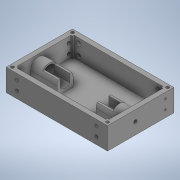
# Autodesk Inventor part: BodyWedgeBaseV3.1
Saved by Autodesk Inventor 2020 (Build 240168000, 168)
## iProperties
Created: 2023-11-26
Part Number: BodyWedgeBaseV3.1
Material: H TPU
Document SubType Name: Modeling
Designer: smz3rm
Density: 0.941117 g/cm^3
Appearance: Generic
Mass: 101.073 g
Surface Area: 496.603 cm^2
Volume: 107.397 cm^3
SideThickness: 6.000 mm
BaseThickness: 3.000 mm
TopThickness: 1.778 mm
BoxWidth: 130.000 mm
BoxLength: 85.000 mm
Height: 30.000 mm
DriveMotorHeight: 15.000 mm
DriveMotorMountThickness: 2.000 mm
DriveMotorOffset: 49.500 mm
DriveMotorDia: 16.500 mm
SideArmorWidth: 15.000 mm
ForkLength: 80.000 mm
WheelWidth: 16.510 mm
DriveMotorHoleDia: 4.200 mm
ForkPlugDia: 4.000 mm
ForkPlugTolerance: 0.750 mm
ForkPlugLength: 8.000 mm
M2ScrewInsertDia: 2.900 mm
M2ScrewInsertDepth: 7.000 mm
M3ScrewHeadDia: 6.100 mm
M3ScrewDia: 3.100 mm
M3ScrewHeadDepth: 2.300 mm
M3ScrewInsertDia: 4.000 mm
M3ScrewInsertDepth: 7.000 mm
M2ScrewHeadDia: 4.000 mm
M2ScrewHeadDepth: 2.200 mm
M2ScrewDia: 2.200 mm
M3ScrewInsertBrim: 8.000 mm
ForkScrewOffset: 8.000 mm
SideScrewVerticalOffset: 6.000 mm
RearScrewHorizontalOffset: 14.000 mm
SideScrewHorizontalOffset: 11.000 mm
M3ScrewHeadTaper: -32.50 deg
Author: smz3rm
Autodesk Inventor part; units mm, degrees
ref_plane "YZ Plane" through (0, 0, 0) normal (1, 0, 0) x (0, 1, 0)
ref_plane "XZ Plane" through (0, 0, 0) normal (0, 1, 0) x (-1, 0, 0)
ref_plane "XY Plane" through (0, 0, 0) normal (0, 0, 1) x (1, 0, 0)
sketch "Sketch1" plane through (0, 0, 0) normal (0, 1, 0) x (-1, 0, 0)
  line L0 (65, 42.5) -> (-65, 42.5)
  line L1 (-65, 42.5) -> (-65, -42.5)
  line L2 (-65, -42.5) -> (65, -42.5)
  line L3 (65, -42.5) -> (65, 42.5)
  line L4 (65, 42.5) -> (-65, -42.5) construction
  line L5 (-65, 42.5) -> (65, -42.5) construction
  line L6 (0, -56) -> (0, 56) projected
  point P0 (0, 0)
  dimension "d0" = 130
  dimension "d1" = 85
  constraints: 12 end point, 2 midpoint, 2 parallel, 1 horizontal, 1 perpendicular
  measures "d0" distance of L2.end L1.end
  measures "d1" distance of L1.end L0.end
sketch "Sketch1 outline for Extrusion1" plane through (0, 0, 0) normal (0, 1, 0) x (-1, 0, 0)
  line L0 (65, -42.5) -> (65, 42.5)
  line L1 (-65, -42.5) -> (65, -42.5)
  line L2 (-65, 42.5) -> (-65, -42.5)
  line L3 (65, 42.5) -> (-65, 42.5)
extrude "Extrusion1" add sketch "Sketch1 outline for Extrusion1" along normal blind 3
sketch "Sketch2" plane through (0, 3, 0) normal (0, 1, 0) x (1, 0, 0)
  line L0 (-65, 42.5) -> (-65, -42.5) projected
  line L1 (-65, -42.5) -> (65, -42.5) projected
  line L2 (65, -42.5) -> (65, 42.5) projected
  line L3 (59, -36.5) -> (-59, -36.5)
  line L4 (-59, -36.5) -> (-59, 36.5)
  line L5 (-59, 36.5) -> (59, 36.5)
  line L6 (59, 36.5) -> (59, -36.5)
  line L7 (59, -36.5) -> (-59, 36.5) construction
  line L8 (-59, -36.5) -> (59, 36.5) construction
  line L9 (65, 42.5) -> (-65, 42.5) projected
  line L10 (-65, -42.5) -> (65, -42.5) projected
  line L11 (65, -42.5) -> (57, -42.5)
  line L12 (57, -42.5) -> (57, -34.5)
  line L13 (57, -34.5) -> (65, -34.5)
  line L14 (65, -34.5) -> (65, -42.5)
  line L15 (-65, -42.5) -> (-57, -42.5)
  line L16 (-57, -42.5) -> (-57, -34.5)
  line L17 (-57, -34.5) -> (-65, -34.5)
  line L18 (-65, -34.5) -> (-65, -42.5)
  line L19 (65, 42.5) -> (-65, 42.5) projected
  line L20 (-65, 42.5) -> (-57, 42.5)
  line L21 (-57, 42.5) -> (-57, 34.5)
  line L22 (-57, 34.5) -> (-65, 34.5)
  line L23 (-65, 34.5) -> (-65, 42.5)
  line L24 (65, 42.5) -> (57, 42.5)
  line L25 (57, 42.5) -> (57, 34.5)
  line L26 (57, 34.5) -> (65, 34.5)
  line L27 (65, 34.5) -> (65, 42.5)
  point P0 (0, 0)
  point P1 (59, 34.5)
  point P2 (57, 36.5)
  point P3 (-59, 34.5)
  point P4 (-57, 36.5)
  point P5 (-59, -34.5)
  point P6 (-57, -36.5)
  point P7 (59, -34.5)
  point P8 (57, -36.5)
  dimension "d36" = 118
  dimension "d37" = 73
  dimension "d173" = 8
  dimension "d176" = 8
  dimension "d177" = 8
  dimension "d178" = 8
  constraints: 44 end point, 10 parallel, 9 perpendicular, 5 horizontal, 2 midpoint
  measures "d36" distance of L4.end L5.end
  measures "d37" distance between parallel lines of L5 L3
  measures "d173" distance of L12.end L13.end
  measures "d176" distance of L15.end L16.end
  measures "d177" distance of L21.end L22.end
  measures "d178" distance of L25.end L26.end
sketch "Sketch2 outline for Extrusion2" plane through (0, 3, 0) normal (0, 1, 0) x (1, 0, 0)
  line L0 (65, 42.5) -> (-65, 42.5)
  line L1 (-65, 42.5) -> (-65, -42.5)
  line L2 (-65, -42.5) -> (65, -42.5)
  line L3 (65, -42.5) -> (65, 42.5)
  line L4 (59, 34.5) -> (59, -34.5)
  line L5 (59, -34.5) -> (57, -34.5)
  line L6 (57, -34.5) -> (57, -36.5)
  line L7 (57, -36.5) -> (-57, -36.5)
  line L8 (-57, -36.5) -> (-57, -34.5)
  line L9 (-57, -34.5) -> (-59, -34.5)
  line L10 (-59, -34.5) -> (-59, 34.5)
  line L11 (-59, 34.5) -> (-57, 34.5)
  line L12 (-57, 34.5) -> (-57, 36.5)
  line L13 (-57, 36.5) -> (57, 36.5)
  line L14 (57, 36.5) -> (57, 34.5)
  line L15 (57, 34.5) -> (59, 34.5)
extrude "Extrusion2" add sketch "Sketch2 outline for Extrusion2" along normal blind 25.222
sketch "Sketch7" plane through (-59, 3, 36.5) normal (1, 0, 0) x (0, 0, -1)
  circle A0 centre (29.5, 12) radius 8.25
  line L0 (79, -3) -> (-6, -3) projected
  circle A1 centre (29.5, 12) radius 10.25
  line L1 (19.25, 12) -> (39.75, 12)
  line L2 (39.75, 12) -> (39.75, 0)
  line L3 (-6, -3) -> (-6, 25.222) projected
  line L4 (19.25, 12) -> (19.25, 0)
  line L5 (71, 0) -> (2, 0) projected
  line L6 (79, -3) -> (-6, -3) projected
  line L7 (-6, -3) -> (-6, 25.222) projected
  line L8 (79, 25.222) -> (-6, 25.222) projected
  line L9 (79, -3) -> (79, 25.222) projected
  line L10 (79, -3) -> (79, 25.222) projected
  point P0 (36.5, -3)
  point P1 (0, 0)
  point P2 (54, -3)
  point P3 (68, 0)
  point P4 (21.25, 12)
  point P5 (37.75, 12)
  dimension "MotorDiameter" = 16.5
  dimension "d18" = 15
  dimension "d20" = 2
  dimension "d183" = 49.5
  constraints: 6 end point, 2 centre point, 2 point on circle, 2 vertical, 1 horizontal, 1 point on line, 1 tangent
  measures "MotorDiameter" diameter of A0
  measures "d18" distance from line of L0 A0.centre
  measures "d20" radial gap between concentric circles of A0 A1
  measures "d183" distance from line of L10 A0.centre
sketch "Sketch7 outline for Extrusion5" plane through (-59, 3, 36.5) normal (1, 0, 0) x (0, 0, -1)
  circle A0 centre (29.5, 12) radius 8.25
  arc A1 (39.75, 12) -> (19.25, 12) centre (29.5, 12) ccw
  line L0 (19.25, 12) -> (19.25, 0)
  line L1 (19.25, 0) -> (39.75, 0)
  line L2 (39.75, 0) -> (39.75, 12)
extrude "Extrusion5" add sketch "Sketch7 outline for Extrusion5" along normal blind 14
sketch "Sketch8" plane through (-45, 3, 36.5) normal (1, 0, 0) x (0, 0, -1)
  arc A0 (39.75, 12) -> (19.25, 12) centre (29.5, 12) ccw
  arc A1 (39.75, 12) -> (19.25, 12) centre (29.5, 12) ccw
  arc A2 (21.25, 12) -> (21.25, 12) centre (29.5, 12) ccw
  line L0 (39.75, 0) -> (19.25, 0)
  circle A3 centre (29.5, 12) radius 7.75
  line L1 (23.4, 17.554503) -> (23.4, 0)
  line L2 (29.5, 19.75) -> (29.5, 4.25)
  line L3 (35.6, 17.554503) -> (35.6, 0)
  circle A4 centre (29.5, 12) radius 8.25
  arc A5 (39.75, 12) -> (19.25, 12) centre (29.5, 12) ccw
  line L4 (35.6, 17.554503) -> (38.114523, 17.554503)
  line L5 (23.4, 17.554503) -> (20.885477, 17.554503)
  line L6 (19.25, 12) -> (19.25, 0)
  line L7 (39.75, 0) -> (19.25, 0)
  line L8 (39.75, 0) -> (39.75, 12)
  line L9 (19.25, 12) -> (19.25, 0)
  line L10 (39.75, 0) -> (19.25, 0)
  line L11 (39.75, 0) -> (39.75, 12)
  point P0 (36.5, -3)
  point P1 (19.25, 12)
  point P2 (44.75, 12)
  point P3 (35.6, 7.219571)
  point P4 (23.4, 7.219571)
  point P5 (20.885477, 17.554503)
  point P6 (39.75, 12)
  point P7 (35.6, 16.780429)
  point P8 (23.4, 16.780429)
  point P9 (19.25, 12)
  point P10 (19.25, 0)
  dimension "d145" = 15.5
  dimension "d146" = 15.5
  dimension "d147" = 12.2
  constraints: 10 end point, 4 point on circle, 2 horizontal, 2 symmetric about line, 1 centre point, 1 coincident, 1 perpendicular, 1 vertical, 2 other
  measures "d145" diameter of A3
  measures "d146" distance of L2.start L2.end
  measures "d147" distance between parallel lines of L1 L3
sketch "Sketch8 outline for Extrusion6" plane through (-45, 3, 36.5) normal (1, 0, 0) x (0, 0, -1)
  line L0 (39.75, 0) -> (39.75, 12)
  arc A0 (39.75, 12) -> (38.114523, 17.554503) centre (29.5, 12) ccw
  line L1 (38.114523, 17.554503) -> (35.6, 17.554503)
  line L2 (35.6, 17.554503) -> (35.6, 7.219571)
  arc A1 (35.6, 7.219571) -> (23.4, 7.219571) centre (29.5, 12) cw
  line L3 (23.4, 7.219571) -> (23.4, 17.554503)
  line L4 (23.4, 17.554503) -> (20.885477, 17.554503)
  arc A2 (20.885477, 17.554503) -> (19.25, 12) centre (29.5, 12) ccw
  line L5 (19.25, 12) -> (19.25, 0)
  line L6 (19.25, 0) -> (39.75, 0)
extrude "Extrusion6" add sketch "Sketch8 outline for Extrusion6" along normal blind 20
sketch "Sketch9" plane through (-59, 17, 13) normal (1, 0, 0) x (0, 0, -1)
  line L0 (55.5, -17) -> (-29.5, -17)
  line L1 (-29.5, -17) -> (-29.5, 11.222)
  arc A0 (-0.1, 3.554503) -> (12.1, 3.554503) centre (6, -2) ccw
  circle A1 centre (6, -2) radius 8.25
  circle A2 centre (6, -2) radius 2.1
  arc A3 (12.1, 3.554503) -> (-0.1, 3.554503) centre (6, -2) ccw
  point P0 (13, -17)
  point P1 (44, -20)
  dimension "d148" = 4.2
  constraints: 1 centre point, 1 coincident, 1 other
  measures "d148" diameter of A2
sketch "Sketch9 outline for Extrusion7" plane through (-59, 17, 13) normal (1, 0, 0) x (0, 0, -1)
  circle A0 centre (6, -2) radius 2.1
extrude "Extrusion7" cut sketch "Sketch9 outline for Extrusion7" against normal up to surface (6 mm away)
mirror "Mirror2" about plane through (0, 0, 0) normal (1, 0, 0) of "Extrusion7", "Extrusion6", "Extrusion5"
sketch "Sketch28" plane through (-59, 3, -36.5) normal (0, 0, 1) x (1, 0, 0)
  line L0 (116, 0) -> (2, 0) projected
  line L1 (110, 19) -> (110, 5)
  line L2 (110, 5) -> (8, 5)
  line L3 (8, 5) -> (8, 19)
  line L4 (8, 19) -> (110, 19)
  circle A0 centre (8, 19) radius 3.05
  circle A1 centre (8, 5) radius 3.05
  circle A2 centre (110, 19) radius 3.05
  circle A3 centre (110, 5) radius 3.05
  line L5 (2, 25.222) -> (116, 25.222) projected
  line L6 (116, 0) -> (116, 25.222) projected
  line L7 (2, 0) -> (2, 25.222) projected
  line L8 (0, 0) -> (0, 25.222) projected
  line L9 (0, 0) -> (0, 25.222) projected
  line L10 (118, 0) -> (118, 25.222) projected
  line L11 (118, 0) -> (118, 25.222) projected
  line L12 (0, 14.1) -> (0, 9.9) projected
  line L13 (118, 9.9) -> (118, 14.1) projected
  line L14 (0, 12) -> (0, 12) projected
  line L15 (118, 12) -> (118, 12) projected
  line L16 (0, 0) -> (0, 12) projected
  line L17 (0, 12) -> (0, 0) projected
  line L18 (118, 12) -> (118, 0) projected
  line L19 (118, 0) -> (118, 12) projected
  point P0 (59, -3)
  point P1 (0, 22.25)
  point P2 (0, 1.75)
  point P3 (118, 22.25)
  point P4 (118, 1.75)
  dimension "d120" = 6.1
  dimension "d121" = 6.1
  dimension "d122" = 6.1
  dimension "d123" = 6.1
  dimension "d132" = 6.222
  dimension "d133" = 5
  dimension "d179" = 8
  dimension "d180" = 8
  constraints: 8 end point, 4 centre point, 4 coincident
  measures "d120" diameter of A0
  measures "d121" diameter of A1
  measures "d122" diameter of A2
  measures "d123" diameter of A3
  measures "d132" distance between parallel lines of L5 L4
  measures "d133" distance between parallel lines of L0 L2
  measures "d179" distance between parallel lines of L9 L3
  measures "d180" distance between parallel lines of L10 L1
sketch "Sketch28 outline for Extrusion24" plane through (-59, 3, -36.5) normal (0, 0, 1) x (1, 0, 0)
  circle A0 centre (110, 5) radius 3.05
  circle A1 centre (110, 19) radius 3.05
  circle A2 centre (8, 5) radius 3.05
  circle A3 centre (8, 19) radius 3.05
extrude "Extrusion24" cut sketch "Sketch28 outline for Extrusion24" against normal blind 2.3 draft -32.5
sketch "Sketch29" plane through (-51, 22, -38.8) normal (0, 0, 1) x (1, 0, 0)
  circle A0 centre (0, 0) radius 1.584738
  circle A1 centre (0, -14) radius 1.584738
  circle A2 centre (102, 0) radius 1.584738
  circle A3 centre (102, -14) radius 1.584738
  circle A4 centre (0, 0) radius 1.55
  circle A5 centre (0, -14) radius 1.55
  circle A6 centre (102, 0) radius 1.55
  circle A7 centre (102, -14) radius 1.584738
  circle A8 centre (102, -14) radius 1.55
  point P0 (51, -22)
  dimension "d126" = 3.1
  dimension "d127" = 3.1
  dimension "d128" = 3.1
  dimension "d129" = 3.1
  constraints: 4 centre point, 4 coincident
  measures "d126" diameter of A4
  measures "d127" diameter of A5
  measures "d128" diameter of A6
  measures "d129" diameter of A8
sketch "Sketch29 outline for Extrusion25" plane through (-51, 22, -38.8) normal (0, 0, 1) x (1, 0, 0)
  circle A0 centre (102, -14) radius 1.55
  circle A1 centre (102, 0) radius 1.55
  circle A2 centre (0, -14) radius 1.55
  circle A3 centre (0, 0) radius 1.55
extrude "Extrusion25" cut sketch "Sketch29 outline for Extrusion25" against normal up to surface (3.7 mm away)
sketch "Sketch30" plane through (0, 28.222, 0) normal (0, 1, 0) x (1, 0, 0)
  line L0 (-65, 42.5) -> (-65, -42.5) projected
  line L1 (65, 42.5) -> (-65, 42.5) projected
  line L2 (-65, -42.5) -> (65, -42.5) projected
  circle A0 centre (-61, 38.5) radius 1.9
  circle A1 centre (-61, -38.5) radius 1.9
  line L3 (-59, 34.5) -> (-57, 34.5) projected
  line L4 (-57, 34.5) -> (-57, 42.5)
  line L5 (65, 42.5) -> (-65, 42.5) projected
  line L6 (-57, 34.5) -> (-65, 34.5)
  line L7 (-57, 34.5) -> (-65, 42.5)
  line L8 (-65, 34.5) -> (-57, 42.5)
  line L9 (-57, -36.5) -> (-57, -34.5) projected
  line L10 (-57, -34.5) -> (-65, -34.5)
  line L11 (-57, -34.5) -> (-57, -42.5)
  line L12 (-65, -42.5) -> (-57, -34.5)
  line L13 (-57, -42.5) -> (-65, -34.5)
  point P0 (0, 0)
  dimension "d139" = 3.8
  constraints: 16 end point, 4 perpendicular, 4 point on line, 2 centre point, 2 coincident, 2 midpoint, 1 equal radius, 1 horizontal
  measures "d139" diameter of A1
sketch "Sketch30 outline for Extrusion26" plane through (0, 28.222, 0) normal (0, 1, 0) x (1, 0, 0)
  circle A0 centre (-61, -38.5) radius 1.9
  circle A1 centre (-61, 38.5) radius 1.9
extrude "Extrusion26" cut sketch "Sketch30 outline for Extrusion26" against normal blind 7
mirror "Mirror11" about plane through (0, 0, 0) normal (1, 0, 0) of "Extrusion26"
sketch "Sketch31" plane through (59, 3, 36.5) normal (-1, 0, 0) x (0, 0, 1)
  line L0 (-39.75, 0) -> (-71, 0) projected
  line L1 (-71, 25.222) -> (-2, 25.222) projected
  line L2 (-71, 25.222) -> (-2, 25.222) projected
  line L3 (-68, 25.222) -> (-68, 0)
  line L4 (-2, 0) -> (-71, 0) projected
  line L5 (-68, 0) -> (-68, 25.4125) projected
  circle A0 centre (-68, 18) radius 2
  circle A1 centre (-68, 6) radius 2
  line L6 (-2, 0) -> (-2, 25.222) projected
  line L7 (-71, 0) -> (-71, 25.222) projected
  line L8 (-79, -3) -> (-79, 25.222) projected
  circle A2 centre (-29.5, 12) radius 2.1 projected
  arc A3 (-19.25, 12) -> (-39.75, 12) centre (-29.5, 12) ccw projected
  line L9 (-19.25, 12) -> (-19.25, 0) projected
  line L10 (-2, 0) -> (-19.25, 0) projected
  line L11 (-39.75, 0) -> (-39.75, 12) projected
  point P0 (-36.5, -3)
  point P1 (0, 25.4125)
  dimension "d152" = 4
  dimension "d153" = 7.222
  dimension "d154" = 4
  dimension "d182" = 11
  constraints: 3 point on line, 2 centre point, 2 end point, 1 vertical, 2 other
  measures "d152" diameter of A0
  measures "d153" distance of L3.start A0.centre
  measures "d154" diameter of A1
  measures "d182" distance between parallel lines of L8 L3
sketch "Sketch31 outline for Extrusion27" plane through (59, 3, 36.5) normal (-1, 0, 0) x (0, 0, 1)
  circle A0 centre (-68, 6) radius 2
  circle A1 centre (-68, 18) radius 2
extrude "Extrusion27" cut sketch "Sketch31 outline for Extrusion27" against normal blind 2.2
sketch "Sketch32" plane through (61.2, 21, -31.5) normal (-1, 0, 0) x (0, 0, 1)
  circle A0 centre (0, 0) radius 2 projected
  circle A1 centre (0, 0) radius 2 projected
  circle A2 centre (0, -12) radius 2 projected
  circle A3 centre (0, -12) radius 2 projected
  circle A4 centre (0, 0) radius 1.1
  circle A5 centre (0, -12) radius 1.1
  point P0 (31.5, -21)
  dimension "d158" = 2.2
  dimension "d159" = 2.2
  constraints: 2 centre point, 2 coincident
  measures "d158" diameter of A4
  measures "d159" diameter of A5
sketch "Sketch32 outline for Extrusion28" plane through (61.2, 21, -31.5) normal (-1, 0, 0) x (0, 0, 1)
  circle A0 centre (0, -12) radius 1.1
  circle A1 centre (0, 0) radius 1.1
extrude "Extrusion28" cut sketch "Sketch32 outline for Extrusion28" against normal up to surface (3.8 mm away)
sketch "Sketch33" plane through (59, 3, 36.5) normal (0, 0, -1) x (-1, 0, 0)
  line L0 (116, 0) -> (2, 0) projected
  line L1 (2, 25.222) -> (116, 25.222) projected
  line L2 (2, 25.222) -> (116, 25.222) projected
  line L3 (8, 25.222) -> (8, 0)
  line L4 (116, 0) -> (2, 0) projected
  circle A0 centre (8, 18) radius 2
  circle A1 centre (8, 6) radius 2
  line L5 (116, 0) -> (116, 25.222) projected
  line L6 (2, 0) -> (2, 25.222) projected
  line L7 (-6, -3) -> (-6, 25.222) projected
  point P0 (59, -3)
  point P1 (0, 0)
  point P2 (108, 0)
  point P3 (108, 25.4125)
  point P4 (0, 25.4125)
  dimension "d163" = 4
  dimension "d164" = 4
  dimension "d165" = 7.222
  dimension "d166" = 6
  dimension "d181" = 14
  constraints: 3 point on line, 2 centre point, 2 end point, 1 perpendicular, 2 other
  measures "d163" diameter of A0
  measures "d164" diameter of A1
  measures "d165" distance of A0.centre L3.start
  measures "d166" distance of L3.end A1.centre
  measures "d181" distance between parallel lines of L7 L3
sketch "Sketch33 outline for Extrusion29" plane through (59, 3, 36.5) normal (0, 0, -1) x (-1, 0, 0)
  circle A0 centre (8, 6) radius 2
  circle A1 centre (8, 18) radius 2
extrude "Extrusion29" cut sketch "Sketch33 outline for Extrusion29" against normal through all
mirror "Mirror13" about plane through (0, 0, 0) normal (1, 0, 0) of "Extrusion27", "Extrusion28", "Extrusion29"
equation "\"d0\" = BoxWidth"
equation "\"d1\" = BoxLength"
equation "\"d2\" = BaseThickness"
equation "\"d37\" = BoxLength - 2 * SideThickness"
equation "\"d18\" = DriveMotorHeight"
equation "\"d20\" = DriveMotorMountThickness"
equation "\"SideThickness\" = 6"
equation "\"BaseThickness\" = 3"
equation "\"TopThickness\" = 1.778"
equation "\"BoxWidth\" = 130"
equation "\"BoxLength\" = 85"
equation "\"Height\" = 30"
equation "\"DriveMotorHeight\" = 0.5 * Height"
equation "\"DriveMotorMountThickness\" = 2"
equation "\"M2ScrewInsertDia\" = 2.9"
equation "\"M2ScrewInsertDepth\" = 7"
equation "\"M3ScrewHeadDia\" = 6.1"
equation "\"M3ScrewDia\" = 3.1"
equation "\"M3ScrewHeadDepth\" = 2.3"
equation "\"DriveMotorOffset\" = 49.5"
equation "\"DriveMotorDia\" = 16.5"
equation "\"SideArmorWidth\" = 15"
equation "\"ForkLength\" = 80"
equation "\"WheelWidth\" = 16.51"
equation "\"DriveMotorHoleDia\" = 4.2"
equation "\"ForkPlugDia\" = 4"
equation "\"ForkPlugTolerance\" = 0.75"
equation "\"ForkPlugLength\" = 8"
equation "\"SideScrewVerticalOffset\" = 6"
equation "\"M3ScrewInsertDia\" = 4"
equation "\"M3ScrewInsertDepth\" = 7"
equation "\"M2ScrewHeadDia\" = 4"
equation "\"M2ScrewHeadDepth\" = 2.2"
equation "\"M2ScrewDia\" = 2.2"
equation "\"M3ScrewInsertBrim\" = 8"
equation "\"ForkScrewOffset\" = 8"
equation "\"RearScrewHorizontalOffset\" = 14"
equation "\"SideScrewHorizontalOffset\" = 11"
equation "\"M3ScrewHeadTaper\" = -32.5deg"
body "Solid1"
